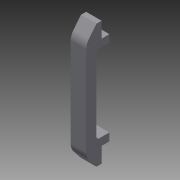
# Autodesk Inventor part: 27080914ServoMount
Saved by Autodesk Inventor 2015 (Build 190159000, 159)
## iProperties
Created: 2013-08-02
Part Number: 27080914ServoMount
Material: Generic
Document SubType Name: Modeling
Designer: Eric
Density: 1 g/cm^3
Appearance: Default
Author: Eric
Autodesk Inventor part; units mm, degrees
ref_plane "YZ Plane" through (0, 0, 0) normal (1, 0, 0) x (0, 1, 0)
ref_plane "XZ Plane" through (0, 0, 0) normal (0, 1, 0) x (-1, 0, 0)
ref_plane "XY Plane" through (0, 0, 0) normal (0, 0, 1) x (1, 0, 0)
sketch "Sketch1" plane through (0, 0, 0) normal (1, 0, 0) x (0, 1, 0)
  line L0 (30, 0) -> (33, 0)
  line L1 (33, 0) -> (33, 3)
  line L2 (33, 3) -> (39, 3)
  line L3 (-9, 3) -> (-3, 3)
  line L4 (-3, 3) -> (-3, 0)
  line L5 (-3, 0) -> (0, 0)
  line L6 (0, 0) -> (0, 4)
  line L7 (1, 5) -> (29, 5)
  line L8 (30, 4) -> (30, 0)
  arc A0 (1, 5) -> (0, 4) centre (1, 4) ccw
  arc A1 (30, 4) -> (29, 5) centre (29, 4) ccw
  line L9 (-4, 9) -> (34, 9)
  line L10 (34, 9) -> (39, 5)
  line L11 (39, 5) -> (39, 3)
  line L12 (-9, 3) -> (-9, 5)
  line L13 (-9, 5) -> (-4, 9)
  point P0 (0, 0)
  point P1 (0, 5)
  point P2 (30, 5)
  point P3 (15, 9)
  point P4 (15, 5)
  dimension "d1" = 3
  dimension "d4" = 30
  dimension "d5" = 2
  dimension "d7" = 3
  dimension "d30" = 38
  dimension "d31" = 4
  dimension "d32" = 2
  dimension "d33" = 2
  dimension "d36" = 3
  dimension "d37" = 3
  dimension "d41" = 6
  dimension "d42" = 6
  constraints: 28 end point, 4 perpendicular, 4 point on circle, 4 point on line, 4 tangent, 3 horizontal, 2 centre point, 2 coincident, 2 midpoint, 2 parallel, 2 vertical, 1 equal radius, 1 horizontal alignment, 1 vertical alignment
  measures "d1" distance of L3.end L4.end
  measures "d4" distance between parallel lines of L8 L6
  measures "d5" distance between parallel lines of L7 L3
  measures "d7" distance of L0.end L1.end
  measures "d30" distance of L9.start L9.end
  measures "d31" distance between parallel lines of L7 L9
  measures "d32" distance of L3.start L12.end
  measures "d33" distance of L10.end L2.end
  measures "d36" distance of L5.end L4.end
  measures "d37" distance of L0.start L0.end
  measures "d41" distance of L3.start L3.end
  measures "d42" distance of L1.end L2.end
extrude "Extrusion1" add sketch "Sketch1" along normal blind 6
fillet "Fillet1" radius 5 2 edges at (3, -4, 9) (3, 34, 9)
body "Solid1"
